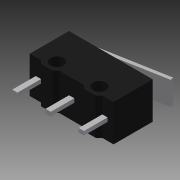
# Autodesk Inventor part: switch
Saved by Autodesk Inventor 2013 (Build 170138000, 138)
## iProperties
Shininess: 41.0
Created: 2014-04-06
Part Number: switch
Document SubType Name: Modeling
Designer: Noa Izumi
Material: Default
Density: 1 g/cm^3
Density: 0.0
Volumn: 0.0
Area: 0.0
PropertySet Name: Model Information
Control State: 0
Master: False
Checked Out: False
Author: Noa Izumi
Autodesk Inventor part; units mm, degrees
ref_plane "YZ Plane" through (0, 0, 0) normal (1, 0, 0) x (0, 1, 0)
ref_plane "XZ Plane" through (0, 0, 0) normal (0, 1, 0) x (-1, 0, 0)
ref_plane "XY Plane" through (0, 0, 0) normal (0, 0, 1) x (1, 0, 0)
sketch "Sketch1" plane through (0, 0, 0) normal (0, 0, 1) x (1, 0, 0)
  line L0 (0, 0) -> (12.8, 0)
  line L1 (12.8, 0) -> (12.8, 6.5)
  line L2 (12.8, 6.5) -> (0, 6.5)
  line L3 (0, 6.5) -> (0, 0)
  dimension "d0" = 12.8
  dimension "d1" = 6.5
  constraints: 8 end point, 2 parallel, 1 horizontal, 1 perpendicular
  measures "d0" distance of L0.start L0.end
  measures "d1" distance of L2.end L0.start
extrude "Extrusion1" add sketch "Sketch1" along normal blind 5.6
sketch "Sketch2" plane through (0, 0, 5.6) normal (0, 0, 1) x (1, 0, 0)
  line L0 (0, 0) -> (0, 6.5) projected
  line L1 (12.8, 0) -> (0, 0) projected
  point P0 (3.15, 1.5)
  point P1 (9.65, 1.5)
  dimension "d4" = 6.5
  dimension "d5" = 3.15
  dimension "d6" = 1.5
  measures "d4" distance of point (9.65, 1.5) point (3.15, 1.5)
  measures "d5" distance from line of L0 point (3.15, 1.5)
  measures "d6" distance from line of L1 point (3.15, 1.5)
hole "Hole1" at (3.15, 1.5, 5.6) at (9.65, 1.5, 5.6) direction (0, 0, -1) diameter 2 end through all
sketch "Sketch3" plane through (0, 0, 5.6) normal (0, 0, 1) x (1, 0, 0)
  line L0 (12.8, 0) -> (0, 0) projected
  line L1 (0, 0) -> (2.225, 0)
  line L2 (2.225, 0) -> (2.225, 0)
  line L3 (1.725, 0.5) -> (0, 0.5)
  line L4 (0, 0.5) -> (0, 0)
  line L5 (4.525, 0.5) -> (8.275, 0.5)
  line L6 (8.775, 0) -> (8.775, 0)
  line L7 (8.775, 0) -> (4.025, 0)
  line L8 (4.025, 0) -> (4.025, 0)
  line L9 (11.075, 0.5) -> (12.8, 0.5)
  line L10 (12.8, 0.5) -> (12.8, 0)
  line L11 (12.8, 0) -> (10.575, 0)
  line L12 (10.575, 0) -> (10.575, 0)
  line L13 (1.725, 0.5) -> (2.225, 0)
  line L14 (4.525, 0.5) -> (4.025, 0)
  line L15 (8.275, 0.5) -> (8.775, 0)
  line L16 (11.075, 0.5) -> (10.575, 0)
  point P0 (2.225, 0.5)
  point P1 (4.025, 0.5)
  point P2 (8.775, 0.5)
  point P3 (10.575, 0.5)
  dimension "d14" = 0.5
  dimension "d17" = 2.225
  dimension "d18" = 2.225
  dimension "d19" = 0.5
  dimension "d20" = 0.5
  dimension "d21" = 0.5
  dimension "d22" = 0.5
  dimension "d23" = 0.5
  dimension "d24" = 0.5
  dimension "d25" = 0.5
  dimension "d26" = 0.5
  dimension "d49" = 1.8
  dimension "d50" = 1.8
  constraints: 32 end point, 10 point on line, 6 parallel, 3 horizontal, 3 perpendicular
  measures "d14" distance of L3.end L0.end
  measures "d17" distance of point (10.575, 0.5) L9.end
  measures "d18" distance of point (2.225, 0.5) L3.end
  measures "d19" distance of L3.start point (2.225, 0.5)
  measures "d20" distance of L2.end point (2.225, 0.5)
  measures "d21" distance of L5.start point (4.025, 0.5)
  measures "d22" distance of L8.end point (4.025, 0.5)
  measures "d23" distance of L5.end point (8.775, 0.5)
  measures "d24" distance of L6.start point (8.775, 0.5)
  measures "d25" distance of L9.start point (10.575, 0.5)
  measures "d26" distance of L12.end point (10.575, 0.5)
  measures "d49" distance of L1.end L7.end
  measures "d50" distance of L11.end L6.end
extrude "Extrusion2" cut sketch "Sketch3" against normal through all
sketch "Sketch4" plane through (0, 6.5, 0) normal (0, 1, 0) x (1, 0, 0)
  line L0 (12.8, 0) -> (0, 0) projected
  line L1 (0, 0) -> (0, -5.6) projected
  line L2 (0.5, -1) -> (1, -1)
  line L3 (1, -1) -> (1, -4.6)
  line L4 (1, -4.6) -> (0.5, -4.6)
  line L5 (0.5, -4.6) -> (0.5, -1)
  dimension "d29" = 3.6
  dimension "d30" = 1
  dimension "d31" = 0.5
  dimension "d32" = 0.5
  constraints: 8 end point, 2 parallel, 1 horizontal, 1 perpendicular
  measures "d29" distance of L4.end L2.start
  measures "d30" distance between parallel lines of L2 L0
  measures "d31" distance between parallel lines of L1 L5
  measures "d32" distance of L3.end L4.end
extrude "Extrusion3" add sketch "Sketch4" along normal blind 0.5
sketch "Sketch5" plane through (0.5, 6.5, 4.6) normal (0, 0, 1) x (1, 0, 0)
  line L0 (0, 0.5) -> (12.6283, 2.79)
  line L1 (0.0892, 0.008) -> (12.7175, 2.298)
  line L2 (12.6283, 2.79) -> (12.7175, 2.298)
  line L3 (0, 0.5) -> (0.0892, 0.008)
  dimension "d35" = 0.5
  constraints: 8 end point, 1 parallel, 1 perpendicular
  measures "d35" distance between parallel lines of L1 L0
extrude "Extrusion4" add sketch "Sketch5" against normal blind 3.6
fillet "Fillet1" radius 0.6 1 edges at (0.5, 7, 2.8)
sketch "Sketch6" plane through (4.525, 0.5, 5.6) normal (0, -1, 0) x (1, 0, 0)
  line L0 (1.475, -2.5) -> (2.275, -2.5)
  line L1 (2.275, -2.5) -> (2.275, -3.1)
  line L2 (2.275, -3.1) -> (1.475, -3.1)
  line L3 (1.475, -3.1) -> (1.475, -2.5)
  line L4 (-3.605, -2.495) -> (-2.805, -2.495)
  line L5 (-2.805, -2.495) -> (-2.805, -3.095)
  line L6 (-2.805, -3.095) -> (-3.605, -3.095)
  line L7 (-3.605, -3.095) -> (-3.605, -2.495)
  line L8 (6.555, -2.495) -> (7.355, -2.495)
  line L9 (7.355, -2.495) -> (7.355, -3.095)
  line L10 (7.355, -3.095) -> (6.555, -3.095)
  line L11 (6.555, -3.095) -> (6.555, -2.495)
  line L12 (-4.525, -5.6) -> (-4.525, 0) projected
  line L13 (0, 0) -> (3.75, 0) projected
  dimension "d39" = 0.6
  dimension "d40" = 0.8
  dimension "d41" = 0.8
  dimension "d42" = 0.8
  dimension "d43" = 4.28
  dimension "d44" = 4.28
  dimension "d45" = 0.92
  dimension "d48" = 2.5
  constraints: 24 end point, 6 parallel, 3 horizontal, 3 perpendicular
  measures "d39" distance of L2.end L0.start
  measures "d40" distance of L0.start L0.end
  measures "d41" distance of L4.start L4.end
  measures "d42" distance of L8.start L8.end
  measures "d43" distance between parallel lines of L3 L5
  measures "d44" distance between parallel lines of L11 L1
  measures "d45" distance between parallel lines of L12 L7
  measures "d48" distance between parallel lines of L0 L13
extrude "Extrusion5" add sketch "Sketch6" along normal blind 3.6
equation "\"d20\" = d19"
equation "\"d21\" = d19"
equation "\"d22\" = d21"
equation "\"d23\" = d19"
equation "\"d24\" = d23"
equation "\"d25\" = d19"
equation "\"d26\" = d25"
